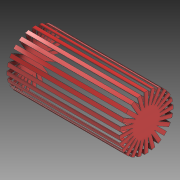
# Autodesk Inventor part: TopRubberBand
Saved by Autodesk Inventor 2021 (Build 250183000, 183)
## iProperties
Created: 2021-04-04
Part Number: TopRubberBand
Material: Generic
Document SubType Name: Modeling
Designer: arybo
Density: 1 g/cm^3
Appearance: Default
Author: arybo
Autodesk Inventor part; units mm, degrees
ref_plane "YZ Plane" through (0, 0, 0) normal (1, 0, 0) x (0, 1, 0)
ref_plane "XZ Plane" through (0, 0, 0) normal (0, 1, 0) x (-1, 0, 0)
ref_plane "XY Plane" through (0, 0, 0) normal (0, 0, 1) x (1, 0, 0)
sketch "Sketch1" plane through (0, 0, 0) normal (0, 0, 1) x (1, 0, 0)
  line L0 (0, 0) -> (149.6822, 0)
  line L1 (149.6822, 0) -> (149.6822, -4.7625)
  line L2 (149.6822, -4.7625) -> (0, -4.7625)
  line L3 (0, -4.7625) -> (0, 0)
  dimension "d0" = 149.6822
  dimension "d1" = 4.7625
  constraints: 8 end point, 1 horizontal, 1 parallel, 1 perpendicular, 1 vertical
  measures "d0" distance of L0.start L0.end
  measures "d1" distance of L0.end L1.end
extrude "Extrusion1" add sketch "Sketch1" along normal blind 0.7937
sketch "Sketch2" plane through (149.6822, -4.7625, 0) normal (1, 0, 0) x (0, 0, -1)
  line L0 (-0.7937, 0) -> (-0.7937, 4.7625) projected
  line L1 (-0.7937, 4.7625) -> (71.5963, 4.7625)
  line L2 (71.5963, 4.7625) -> (71.5963, 0)
  line L3 (71.5963, 0) -> (-0.7937, 0)
  line L4 (-0.7937, 0) -> (-0.7937, 4.7625)
  point P0 (0, 4.7625)
  dimension "d4" = 72.39
  constraints: 8 end point, 2 perpendicular, 1 collinear, 1 horizontal
  measures "d4" distance of L0.end L1.end
extrude "Extrusion2" add sketch "Sketch2" along normal blind 0.7937
sketch "Sketch3" plane through (0, -4.7625, 0) normal (-1, 0, 0) x (0, 0, 1)
  line L0 (0, 4.7625) -> (0.7937, 4.7625) projected
  line L1 (-71.5963, 0) -> (-71.5963, 4.7625) projected
  line L2 (0.7937, 4.7625) -> (-71.5963, 4.7625)
  line L3 (0, 0) -> (-71.5963, 0) projected
  line L4 (-71.5963, 4.7625) -> (-71.5963, 0)
  line L5 (0.7937, 4.7625) -> (0.7937, 0) projected
  line L6 (-71.5963, 0) -> (0.7937, 0)
  line L7 (0.7937, 0) -> (0.7937, 4.7625)
  circle A0 centre (-35.4013, 2.3813) radius 2.2098
  dimension "d7" = 4.4196
  constraints: 8 end point, 3 perpendicular, 1 centre point, 1 horizontal
  measures "d7" diameter of A0
extrude "Extrusion3" add sketch "Sketch3" along normal blind 0.7937
sketch "Sketch4" plane through (149.6822, -4.7625, -71.5963) normal (0, 0, -1) x (-1, 0, 0)
  line L0 (0, 4.7625) -> (149.6822, 4.7625) projected
  line L1 (0, 4.7625) -> (149.6822, 4.7625)
  line L2 (149.6822, 0) -> (0, 0) projected
  line L3 (149.6822, 4.7625) -> (149.6822, 0)
  line L4 (149.6822, 0) -> (0, 0)
  line L5 (0, 0) -> (0, 4.7625) projected
  line L6 (0, 0) -> (0, 4.7625)
  constraints: 8 end point, 2 perpendicular, 1 collinear, 1 horizontal
extrude "Extrusion4" add sketch "Sketch4" against normal blind 0.7937
pattern_circular "Circular Pattern1" count 24 over 360 about axis through (0, -2.3813, -35.4013) along (-1, 0, 0) of "Extrusion4", "Extrusion3", "Extrusion1", "Extrusion2"
body "Solid1"
